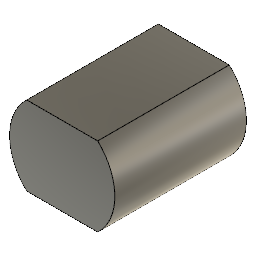
Engine v84 (Autodesk Fusion 360 archive; units mm, degrees)
design "DC  MOTOR"
Autodesk Fusion 360 part; units mm, degrees
sketch "Sketch1" plane through (0, 0, 0) normal (0, 1, 0) x (1, 0, 0)
  line L0 (0, 0) -> (0, -15) construction
  line L1 (0, -15) -> (13.5, -15)
  line L2 (13.5, -15) -> (13.5, 0) construction
  line L3 (13.5, 0) -> (0, 0)
  line L4 (13.5, -7.5) -> (16.75, -7.5) construction
  line L5 (0, -7.5) -> (-3.25, -7.5) construction
  arc A0 (0, 0) -> (0, -15) centre (7.0288, -7.5) ccw
  arc A1 (13.5, -15) -> (13.5, 0) centre (6.4712, -7.5) ccw
  dimension "d1" = 13.5
  dimension "d2" = 3.25
  dimension "d3" = 3.25
  constraint coincident L0.start L3.end
  constraint vertical L0
  constraint perpendicular L0 L1
  constraint perpendicular L1 L2
  constraint perpendicular L0 L3
  constraint midpoint L2 L4.start
  constraint perpendicular L2 L4
  constraint midpoint L0 L5.start
  constraint perpendicular L0 L5
  constraint coincident L5.end A0
  constraint coincident L4.end A1
  measures "d1" distance of L0.end L1.end
  measures "d2" distance of L4.start L4.end
  measures "d3" distance of L5.start L5.end
extrude "Extrude1" add sketch "Sketch1" along normal blind 25
